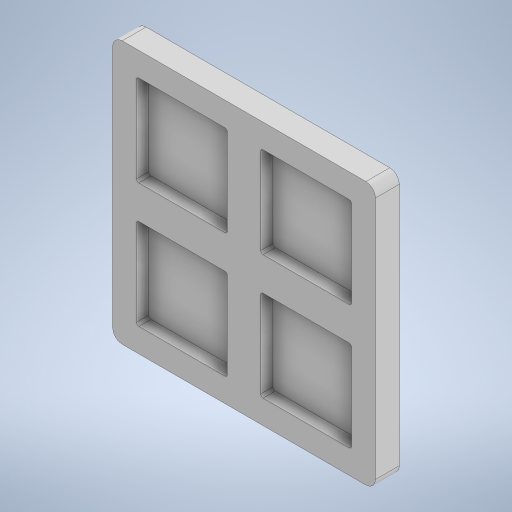
# Autodesk Inventor part: Paletka
Saved by Autodesk Inventor 2023 (Build 270158000, 158)
## iProperties
Created: 2024-01-19
Part Number: Paletka
Material: Všeobecné
Document SubType Name: Modeling
Designer: zak
Density: 1 g/cm^3
Appearance: Výchozí
Author: zak
Autodesk Inventor part; units mm, degrees
ref_plane "YZ Plane" through (0, 0, 0) normal (1, 0, 0) x (0, 1, 0)
ref_plane "XZ Plane" through (0, 0, 0) normal (0, 1, 0) x (-1, 0, 0)
ref_plane "XY Plane" through (0, 0, 0) normal (0, 0, 1) x (1, 0, 0)
sketch "Náčrt2" plane through (0, 0, 0) normal (0, 0, 1) x (1, 0, 0)
  line L0 (-77, 0) -> (77, 0) projected
  line L1 (0, -77) -> (0, 77) projected
  line L2 (-55, 55) -> (55, 55)
  line L3 (55, 55) -> (55, -55)
  line L4 (55, -55) -> (-55, -55)
  line L5 (-55, -55) -> (-55, 55)
  point P0 (0, 0)
  dimension "d0" = 110
  dimension "d1" = 110
  dimension "d2" = 55
  constraints: 8 end point, 2 parallel, 1 horizontal, 1 perpendicular, 1 other
  measures "d0" distance of L3.end L4.end
  measures "d1" distance of L2.end L3.end
  measures "d2" distance between parallel lines of L0 L2
extrude "Vysunutí1" add sketch "Náčrt2" along normal blind 10
sketch "Náčrt3" plane through (0, 0, 10) normal (0, 0, 1) x (1, 0, 0)
  line L0 (-45, 45) -> (-7, 45)
  line L1 (-7, 45) -> (-7, 7)
  line L2 (-7, 7) -> (-45, 7)
  line L3 (-45, 7) -> (-45, 45)
  line L4 (-77, 0) -> (77, 0) projected
  line L5 (0, -77) -> (0, 77) projected
  line L6 (-55, 55) -> (-55, -55) projected
  line L7 (55, 55) -> (-55, 55) projected
  line L8 (7, 45) -> (45, 45)
  line L9 (7, 7) -> (7, 45)
  line L10 (45, 7) -> (7, 7)
  line L11 (45, 45) -> (45, 7)
  line L12 (-45, -7) -> (-7, -7)
  line L13 (-45, -45) -> (-45, -7)
  line L14 (-7, -45) -> (-45, -45)
  line L15 (-7, -7) -> (-7, -45)
  line L16 (7, -7) -> (45, -7)
  line L17 (7, -45) -> (7, -7)
  line L18 (45, -45) -> (7, -45)
  line L19 (45, -7) -> (45, -45)
  point P0 (0, 0)
  dimension "d5" = 38
  dimension "d6" = 38
  dimension "d7" = 10
  dimension "d8" = 10
  dimension "d11" = 52
  dimension "d14" = 52
  constraints: 32 end point, 2 horizontal, 2 parallel, 1 perpendicular, 1 vertical, 24 other
  measures "d5" distance of L1.end L2.end
  measures "d6" distance of L0.end L1.end
  measures "d7" distance between parallel lines of L3 L6
  measures "d8" distance between parallel lines of L7 L0
  measures "d11" distance of L0.start L8.start
  measures "d14" distance of L0.start L12.start
extrude "Vysunutí2" cut sketch "Náčrt3" against normal blind 5 contours L0 L1 L2 L3 | L8 L11 L10 L9 | L12 L15 L14 L13 | L16 L19 L18 L17
fillet "Zaoblení1" radius 1 16 edges at (-45, 45, 7.5) (7, 45, 7.5) (-45, -7, 7.5) (7, -7, 7.5) (45, -45, 7.5) (-7, -45, 7.5) (45, 7, 7.5) (-7, 7, 7.5) (45, 45, 7.5) (-7, 45, 7.5) (45, -7, 7.5) (-7, -7, 7.5) (-45, -45, 7.5) (7, -45, 7.5) (7, 7, 7.5) (-45, 7, 7.5)
fillet "Zaoblení2" radius 4 4 edges at (-55, -55, 5) (55, -55, 5) (55, 55, 5) (-55, 55, 5)
equation "\"d1\" = d0"
equation "\"d2\" = 0.5 * d1"
equation "\"d6\" = d5"
equation "\"d8\" = d7"
equation "\"d14\" = d11"
